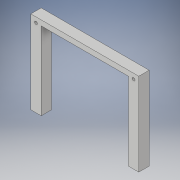
# Autodesk Inventor part: U-Part Gen 2
Saved by Autodesk Inventor 2019 (Build 230136000, 136)
## iProperties
Created: 2019-10-05
Part Number: U-Part Gen 2
Material: Generic
Document SubType Name: Modeling
Designer: Delta
Density: 1 g/cm^3
Appearance: Default
Author: Delta
Autodesk Inventor part; units mm, degrees
ref_plane "YZ Plane" through (0, 0, 0) normal (1, 0, 0) x (0, 1, 0)
ref_plane "XZ Plane" through (0, 0, 0) normal (0, 1, 0) x (-1, 0, 0)
ref_plane "XY Plane" through (0, 0, 0) normal (0, 0, 1) x (1, 0, 0)
sketch "Sketch1" plane through (0, 0, 0) normal (0, 0, 1) x (1, 0, 0)
  line L0 (0, 0) -> (132.08, 0)
  line L1 (132.08, 0) -> (132.08, -6.35)
  line L2 (132.08, -6.35) -> (0, -6.35)
  line L3 (0, -6.35) -> (0, 0)
  line L4 (132.08, 0) -> (119.38, 0)
  line L5 (119.38, 0) -> (119.38, -101.6)
  line L6 (119.38, -101.6) -> (132.08, -101.6)
  line L7 (132.08, -101.6) -> (132.08, 0)
  line L8 (0, 0) -> (12.7, 0)
  line L9 (12.7, 0) -> (12.7, -101.6)
  line L10 (12.7, -101.6) -> (0, -101.6)
  line L11 (0, -101.6) -> (0, 0)
  line L12 (0, -88.9) -> (25.4, -88.9) construction
  line L13 (12.7, -101.6) -> (38.1, -101.6) construction
  dimension "d1" = 6.35
  dimension "d2" = 12.7
  dimension "d3" = 101.6
  dimension "d5" = 101.6
  dimension "d6" = 12.7
  dimension "d13" = 12.7
  dimension "d15" = 106.68
  constraints: 28 end point, 6 parallel, 5 horizontal, 3 perpendicular, 1 point on line
  measures "d1" distance of L0.end L1.end
  measures "d2" distance of L6.end L5.end
  measures "d3" distance of L5.end L4.end
  measures "d5" distance between parallel lines of L10 L0
  measures "d6" distance of L12.start L10.end
  measures "d13" distance between parallel lines of L11 L9
  measures "d15" distance between parallel lines of L5 L9
extrude "Extrusion2" add sketch "Sketch1" along normal blind 12.7
sketch "Sketch3" plane through (0, 0, 12.7) normal (0, 0, 1) x (1, 0, 0)
  line L0 (0, 0) -> (0, -101.6) projected
  line L1 (12.7, -101.6) -> (12.7, -6.35) projected
  line L2 (132.08, 0) -> (0, 0) projected
  line L3 (132.08, -101.6) -> (132.08, 0) projected
  circle A0 centre (6.35, -6.35) radius 1.778
  circle A1 centre (125.73, -6.35) radius 1.778
  dimension "d18" = 6.35
  dimension "d19" = 12.7
  dimension "d20" = 6.35
  dimension "d21" = 6.35
  dimension "d22" = 6.35
  dimension "d23" = 3.556
  dimension "d24" = 3.556
  constraints: 2 centre point, 2 coincident
  measures "d18" distance from line of L0 point (6.35, -6.35)
  measures "d19" distance between parallel lines of L0 L1
  measures "d20" distance from line of L2 point (6.35, -6.35)
  measures "d21" distance from line of L2 point (125.73, -6.35)
  measures "d22" distance from line of L3 point (125.73, -6.35)
  measures "d23" diameter of A0
  measures "d24" diameter of A1
extrude "Extrusion3" cut sketch "Sketch3" against normal blind 25.4
equation "\"d5\" = d3"
equation "\"d6\" = d4"
equation "\"d18\" = 0.5 * d19"
equation "\"d21\" = d20"
equation "\"d22\" = d18"
equation "\"d4\" = d2"
body "Solid2"
